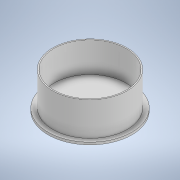
# Autodesk Inventor part: Base Plug
Saved by Autodesk Inventor 2020 (Build 240168000, 168)
## iProperties
Created: 2020-01-07
Part Number: Base Plug
Material: Generic
Document SubType Name: Modeling
Designer: ellio
Density: 1 g/cm^3
Appearance: Default
Author: ellio
Autodesk Inventor part; units mm, degrees
ref_plane "YZ Plane" through (0, 0, 0) normal (1, 0, 0) x (0, 1, 0)
ref_plane "XZ Plane" through (0, 0, 0) normal (0, 1, 0) x (-1, 0, 0)
ref_plane "XY Plane" through (0, 0, 0) normal (0, 0, 1) x (1, 0, 0)
sketch "Sketch1" plane through (0, 0, 0) normal (0, 1, 0) x (-1, 0, 0)
  circle A0 centre (0, 0) radius 57.15
  dimension "d0" = 114.3
  constraints: 1 centre point, 1 coincident
  measures "d0" diameter of A0
extrude "Extrusion1" add sketch "Sketch1" along normal blind 3.175
sketch "Sketch2" plane through (0, 3.175, 0) normal (0, 1, 0) x (1, 0, 0)
  circle A0 centre (0, 0) radius 50.8
  circle A1 centre (0, 0) radius 49.2125
  dimension "d3" = 101.6
  dimension "d4" = 98.425
  constraints: 2 centre point, 2 coincident
  measures "d3" diameter of A0
  measures "d4" diameter of A1
extrude "Extrusion2" add sketch "Sketch2" along normal blind 45.72
sketch "Sketch3" plane through (0, 3.175, 0) normal (0, 1, 0) x (1, 0, 0)
  circle A0 centre (0, 0) radius 49.2125
  constraints: 1 centre point, 1 coincident
extrude "Extrusion3" add sketch "Sketch3" along normal blind 4.7625
sketch "Sketch4" plane through (0, 0, 0) normal (0, -1, 0) x (1, 0, 0)
  line L0 (3.175, 3.175) -> (34.925, 3.175)
  line L1 (34.925, 3.175) -> (34.925, -3.175)
  line L2 (34.925, -3.175) -> (3.175, -3.175)
  line L3 (3.175, -3.175) -> (3.175, -34.925)
  line L4 (3.175, -34.925) -> (-3.175, -34.925)
  line L5 (-3.175, -34.925) -> (-3.175, -3.175)
  line L6 (-3.175, -3.175) -> (-34.925, -3.175)
  line L7 (-34.925, -3.175) -> (-34.925, 3.175)
  line L8 (-34.925, 3.175) -> (-3.175, 3.175)
  line L9 (-3.175, 3.175) -> (-3.175, 34.925)
  line L10 (-3.175, 34.925) -> (3.175, 34.925)
  line L11 (3.175, 34.925) -> (3.175, 3.175)
  point P0 (0, 0)
  dimension "d9" = 31.75
  dimension "d10" = 6.35
  dimension "d11" = 31.75
  dimension "d12" = 6.35
  dimension "d13" = 31.75
  dimension "d14" = 31.75
  constraints: 24 end point, 10 perpendicular, 2 horizontal, 1 point on line
  measures "d9" distance of L0.start L0.end
  measures "d10" distance of L0.end L1.end
  measures "d11" distance of L2.end L3.end
  measures "d12" distance of L3.end L4.end
  measures "d13" distance of L5.end L6.end
  measures "d14" distance of L8.end L9.end
extrude "Extrusion4" cut sketch "Sketch4" against normal blind 6.35
body "Solid1"
